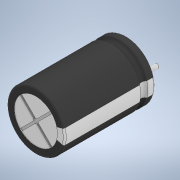
# Autodesk Inventor part: CPOL-D8-H11_5-P3_5
Saved by Autodesk Inventor 2020.1 (Build 241239000, 239)
## iProperties
Created: 2020-03-13
Part Number: CPOL-D8-H11_5-P3_5
Material: Generic
Document SubType Name: Modeling
Designer: yusaku
Density: 1 g/cm^3
Appearance: Default
Author: yusaku
Autodesk Inventor part; units mm, degrees
ref_plane "YZ Plane" through (0, 0, 0) normal (1, 0, 0) x (0, 1, 0)
ref_plane "XZ Plane" through (0, 0, 0) normal (0, 1, 0) x (-1, 0, 0)
ref_plane "XY Plane" through (0, 0, 0) normal (0, 0, 1) x (1, 0, 0)
sketch "Sketch1" plane through (0, 0, 0) normal (0, 1, 0) x (-1, 0, 0)
  line L0 (0, 0) -> (3.8, 0)
  line L1 (4, -0.2) -> (4, -1)
  arc A0 (4, -1) -> (4, -2) centre (4.2887, -1.5) ccw
  line L2 (4, -2) -> (4, -12.3)
  line L3 (3.8, -12.5) -> (0, -12.5)
  line L4 (0, -12.5) -> (0, 0)
  line L5 (4, -1) -> (3.134, -1.5) construction
  arc A1 (3.8, -12.5) -> (4, -12.3) centre (3.8, -12.3) ccw
  arc A2 (4, -0.2) -> (3.8, 0) centre (3.8, -0.2) ccw
  line L6 (0, -12.5) -> (0, -12.51)
  line L7 (0, -12.51) -> (3.8, -12.51)
  arc A3 (3.8, -12.51) -> (4.01, -12.3) centre (3.8, -12.3) ccw
  line L8 (4.01, -12.3) -> (4.01, -1.9942)
  arc A4 (4.01, -1.0058) -> (4.01, -1.9942) centre (4.2887, -1.5) ccw
  line L9 (4.01, -1.0058) -> (4.01, -0.2)
  arc A5 (4.01, -0.2) -> (3.864, 0) centre (3.8, -0.2) ccw
  line L10 (3.864, 0) -> (3.8, 0)
  line L11 (3.7113, -1.5) -> (3.7213, -1.5) construction
  point P0 (4, 0)
  point P1 (4, -12.5)
  dimension "d0" = 4
  dimension "d1" = 12.5
  dimension "d3" = 1
  dimension "d4" = 60
  dimension "d5" = 1
  dimension "d7" = 0.2
  dimension "d8" = 0.2
  dimension "d20" = 0.01
  constraints: 24 end point, 14 point on circle, 8 point on line, 8 tangent, 7 perpendicular, 6 centre point, 3 concentric, 2 horizontal, 1 horizontal alignment, 1 vertical
  measures "d0" distance of L0.start point (4, 0)
  measures "d1" distance between parallel lines of L3 L0
  measures "d3" distance of point (4, 0) L1.end
  measures "d4" angle of L1 L5
  measures "d5" distance of L2.start L1.end
  measures "d7" radius of A1
  measures "d8" radius of A2
  measures "d20" distance between parallel lines of L3 L7
revolve "Revolution1" add sketch "Sketch1" angle 360 about axis through (0, 0, -12.5) along (0, 0, 1) contours L0 A2 L1 A0 L2 A1 L3 L4
revolve "Revolution2" add sketch "Sketch1" angle 30 mid plane about axis through (0, 0, -12.5) along (0, 0, 1) contours L10 A5 L9 A4 L8 A3 L7 L6 L3 A1 L2 A0 L1 A2
sketch "Sketch2" plane through (0, 0, -12.5) normal (0, 0, -1) x (-1, 0, 0)
  circle A0 centre (0, 0) radius 3
  dimension "d9" = 6
  constraints: 1 centre point, 1 coincident
  measures "d9" diameter of A0
extrude "Extrusion1" cut sketch "Sketch2" against normal mid plane 0.1
sketch "Sketch6" plane through (0, 0, 0) normal (0, 0, 1) x (1, 0, 0)
  circle A0 centre (0, 0) radius 3
  dimension "d27" = 6
  constraints: 1 centre point, 1 coincident
  measures "d27" diameter of A0
extrude "Extrusion4" add sketch "Sketch6" along normal blind 0.5
sketch "Sketch3" plane through (0, 0, 0.5) normal (0, 0, 1) x (1, 0, 0)
  circle A0 centre (-1.75, 0) radius 0.3
  circle A1 centre (1.75, 0) radius 0.3
  line L0 (0, -5.6) -> (0, 5.6) construction
  point P0 (0, 0)
  dimension "d12" = 3.5
  dimension "d13" = 0.6
  constraints: 2 centre point, 1 equal radius, 1 horizontal alignment, 1 symmetric about line
  measures "d12" distance of A1.centre A0.centre
  measures "d13" diameter of A0
extrude "Extrusion2" add sketch "Sketch3" along normal blind 2
sketch "Sketch5" plane through (0, 0, -12.45) normal (0, 0, -1) x (-1, 0, 0)
  line L0 (-2.0126, 2.2247) -> (0, 0.2121)
  line L1 (0, 0.2121) -> (2.0126, 2.2247)
  circle A0 centre (0, 0) radius 3 projected
  line L2 (-2.2247, 2.0126) -> (-0.2121, 0)
  line L3 (-0.2121, 0) -> (-2.2247, -2.0126)
  line L4 (-2.0126, -2.2247) -> (0, -0.2121)
  line L5 (0, -0.2121) -> (2.0126, -2.2247)
  line L6 (2.2247, -2.0126) -> (0.2121, 0)
  line L7 (0.2121, 0) -> (2.2247, 2.0126)
  line L8 (0, 0.2121) -> (0.2121, 0) construction
  line L9 (0, -0.2121) -> (-0.2121, 0) construction
  line L10 (-0.2121, 0) -> (0, 0.2121) construction
  line L11 (0, -0.2121) -> (0.2121, 0) construction
  dimension "d23" = 0.3
  constraints: 24 end point, 7 collinear, 2 horizontal alignment, 2 parallel, 2 point on line, 2 vertical alignment, 1 perpendicular, 9 other
  measures "d23" distance between parallel lines of L7 L1
extrude "Extrusion3" cut sketch "Sketch5" against normal blind 0.1 contours L0 L1 A0 L7 L6 L5 L4 L3 L2
fillet "Fillet1" radius 0.2 4 edges at (0, 0.2121, -12.4) (-0.2121, 0, -12.4) (0, -0.2121, -12.4) (0.2121, 0, -12.4)
body "Solid1"
